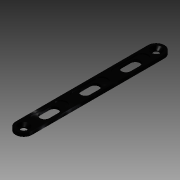
# Autodesk Inventor part: 13_1087_018
Saved by Autodesk Inventor 2014 (Build 180170000, 170)
## iProperties
Created: 2013-09-05
Part Number: 13_1087_018
Material: Allgemein
Document SubType Name: Modeling
Designer: vogel
Density: 1 g/cm^3
Appearance: Schwarz
Author: vogel
Autodesk Inventor part; units mm, degrees
ref_plane "YZ Plane" through (0, 0, 0) normal (1, 0, 0) x (0, 1, 0)
ref_plane "XZ Plane" through (0, 0, 0) normal (0, 1, 0) x (-1, 0, 0)
ref_plane "XY Plane" through (0, 0, 0) normal (0, 0, 1) x (1, 0, 0)
sketch "Skizze1" plane through (0, 0, 0) normal (0, 0, 1) x (1, 0, 0)
  line L0 (-4.9, 0) -> (4.9, 0) projected
  line L1 (0, -44.8) -> (0, 44.8) projected
  line L2 (0, 5) -> (0, -5) construction
  line L3 (2.5, 5) -> (2.5, -5)
  line L4 (-2.5, -5) -> (-2.5, 5)
  arc A0 (2.5, 5) -> (-2.5, 5) centre (0, 5) ccw
  arc A1 (-2.5, -5) -> (2.5, -5) centre (0, -5) ccw
  line L5 (0, 28.5) -> (0, -28.5) construction
  line L6 (-3.5, 28.5) -> (-3.5, -28.5)
  line L7 (3.5, -28.5) -> (3.5, 28.5)
  arc A2 (3.5, 28.5) -> (-3.5, 28.5) centre (0, 28.5) ccw
  arc A3 (-3.5, -28.5) -> (3.5, -28.5) centre (0, -28.5) ccw
  line L8 (0, 12.5) -> (0, 22.5) construction
  line L9 (2.5, 12.5) -> (2.5, 22.5)
  line L10 (-2.5, 22.5) -> (-2.5, 12.5)
  arc A4 (-2.5, 12.5) -> (2.5, 12.5) centre (0, 12.5) ccw
  arc A5 (2.5, 22.5) -> (-2.5, 22.5) centre (0, 22.5) ccw
  line L11 (0, -22.5) -> (0, -12.5) construction
  line L12 (2.5, -22.5) -> (2.5, -12.5)
  line L13 (-2.5, -12.5) -> (-2.5, -22.5)
  arc A6 (-2.5, -22.5) -> (2.5, -22.5) centre (0, -22.5) ccw
  arc A7 (2.5, -12.5) -> (-2.5, -12.5) centre (0, -12.5) ccw
  point P0 (0, 0)
  point P1 (0, 0)
  point P2 (0, 0)
  point P3 (0, 17.5)
  point P4 (0, -17.5)
  dimension "d0" = 5
  dimension "d1" = 15
  dimension "d2" = 7
  dimension "d3" = 10
  dimension "d4" = 10
  dimension "d5" = 32
  dimension "d31" = 2.5
  constraints: 32 end point, 16 point on circle, 16 tangent, 8 centre point, 8 point on line, 4 midpoint, 4 parallel, 2 collinear, 2 equal radius, 2 other
  measures "d0" distance between parallel lines of L3 L4
  measures "d2" distance between parallel lines of L7 L6
  measures "d3" distance edge to line of A7 L0
  measures "d4" distance edge to line of A4 L0
extrude "Extrusion1" add sketch "Skizze1" along normal blind 0.5 contours L6 A2 L1 A5 L10 A4 A0 L4 L0 | L0 L4 A1 L1 A7 L13 A6 A3 L6 | A2 L7 L0 L3 A0 L1 A4 L9 A5 | L1 A6 L12 A7 A1 L3 L0 L7 A3
sketch "Skizze2" plane through (0, 0, 0) normal (0, 0, -1) x (-1, 0, 0)
  line L0 (3.5, 28.5) -> (3.5, -28.5) projected
  arc A0 (3.5, 28.5) -> (-3.5, 28.5) centre (0, 28.5) ccw projected
  line L1 (-3.5, -28.5) -> (-3.5, 28.5) projected
  arc A1 (-3.5, -28.5) -> (3.5, -28.5) centre (0, -28.5) ccw projected
  point P0 (0, 0)
extrude "Extrusion2" add sketch "Skizze2" along normal blind 1
sketch "Skizze3" plane through (0, 0, 0.5) normal (0, 0, 1) x (1, 0, 0)
  arc A0 (-3.5, -28.5) -> (3.5, -28.5) centre (0, -28.5) ccw projected
  arc A1 (3.5, 28.5) -> (-3.5, 28.5) centre (0, 28.5) ccw projected
  point P0 (0, 0)
  constraints: 2 coincident
hole "Bohrung1" at (0, 28.5, 0.5) at (0, -28.5, 0.5) direction (0, 0, -1) diameter 2.4 end through all countersink diameter 4.6 countersink angle 90
sketch "Skizze5" plane through (0, 0, 0) normal (0, 0, 1) x (1, 0, 0)
  arc A0 (-2.5, -22.5) -> (2.5, -22.5) centre (0, -22.5) ccw projected
  line L0 (2.5, -22.5) -> (2.5, -12.5) projected
  arc A1 (2.5, -12.5) -> (-2.5, -12.5) centre (0, -12.5) ccw projected
  line L1 (0, -15.5) -> (0, -19.5) construction
  line L2 (2, -15.5) -> (2, -19.5)
  line L3 (-2, -19.5) -> (-2, -15.5)
  arc A2 (2, -15.5) -> (-2, -15.5) centre (0, -15.5) ccw
  arc A3 (-2, -19.5) -> (2, -19.5) centre (0, -19.5) ccw
  line L4 (0, -22.5) -> (0, -12.5)
  line L5 (0, -12.5) -> (0, -17.5)
  line L6 (-1.3218, -17.5) -> (0, -17.5)
  point P0 (0, 0)
  point P1 (0, -17.5)
  dimension "d24" = 4
  dimension "d25" = 8
  constraints: 14 end point, 4 point on circle, 4 tangent, 3 parallel, 2 centre point, 2 midpoint, 1 coincident, 1 perpendicular
  measures "d24" distance between parallel lines of L2 L3
extrude "Extrusion3" cut sketch "Skizze5" against normal through all
pattern_linear "Rechteckige Anordnung1" count 3 spacing 17.5 along (0, 1, 0) of "Extrusion3"
